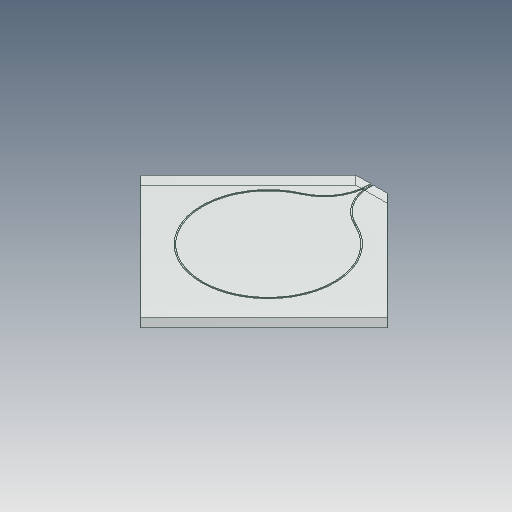
# Autodesk Inventor part: Scintillator Tile
Saved by Autodesk Inventor 2020 (Build 240168000, 168)
## iProperties
Created: 2015-08-14
Part Number: Scintillator Tile
Material: ABS Plastic
Document SubType Name: Modeling
Designer: Cosmic
Density: 1.06 g/cm^3
Appearance: Clear
Author: Cosmic
Autodesk Inventor part; units mm, degrees
note: some values were not read from the file. Chosen so that the rebuilt part matches the saved one: sketch regions of "Extrusion13". Left out: dimensions or parameters whose unit could not be read.
ref_plane "YZ Plane" through (0, 0, 0) normal (1, 0, 0) x (0, 1, 0)
ref_plane "XZ Plane" through (0, 0, 0) normal (0, 1, 0) x (-1, 0, 0)
ref_plane "XY Plane" through (0, 0, 0) normal (0, 0, 1) x (1, 0, 0)
sketch "Sketch11" plane through (0, 0, 0) normal (0, 0, 1) x (1, 0, 0)
  line L0 (0, -141.4214) -> (141.4214, 0)
  line L1 (141.4214, 0) -> (0, 141.4214)
  line L2 (0, 141.4214) -> (-141.4214, 0)
  line L3 (-141.4214, 0) -> (0, -141.4214)
  line L4 (0, -141.4214) -> (0, 141.4214) construction
  line L5 (141.4214, 0) -> (-141.4214, 0) construction
  line L6 (0, -141.4214) -> (200, -141.4214) construction
  point P0 (0, 0)
  dimension "d80" = 200
  dimension "d81" = 45
  dimension "d82" = 200
  constraints: 14 end point, 2 midpoint, 2 parallel, 1 equal length, 1 horizontal, 1 perpendicular
  measures "d80" distance of L0.start L0.end
  measures "d81" angle of L6 L0
  measures "d82" distance of L1.end L0.end
extrude "Extrusion12" add sketch "Sketch11" along normal blind 10
chamfer "Chamfer1" distance 25.4 angle 45 1 edges at (0, 141.4214, 5)
sketch "Sketch13" plane through (0, 0, 10) normal (0, 0, 1) x (1, 0, 0)
  line L0 (72.5, 123.4608) -> (-72.5, 123.4608)
  arc A0 (-30.4632, 73.5832) -> (30.4632, 73.5832) centre (0, 5.0485) ccw
  arc A1 (-30.9912, 74.7711) -> (-38.9161, 70.678) centre (0, 5.0485) ccw
  arc A2 (-30.9912, 74.7711) -> (-1.3, 120.4608) centre (-51.3, 120.4608) ccw
  arc A3 (30.9912, 74.7711) -> (80.4111, 79.8094) centre (51.3, 120.4608) ccw
  arc A4 (-38.9161, 70.678) -> (-30.4632, 73.5832) centre (-51.3, 120.4608) ccw
  arc A5 (22.6429, 77.9114) -> (30.4632, 73.5832) centre (51.3, 120.4608) ccw
  line L1 (-51.3, 120.4608) -> (51.3, 120.4608)
  arc A6 (-80.4111, 79.8094) -> (-30.9912, 74.7711) centre (-51.3, 120.4608) ccw
  arc A7 (-80.3294, 78.1644) -> (-38.9161, 70.678) centre (-51.3, 120.4608) ccw
  arc A8 (-1.3, 120.4608) -> (-80.4111, 79.8094) centre (-51.3, 120.4608) ccw
  arc A9 (-30.4632, 73.5832) -> (-22.6429, 77.9114) centre (-51.3, 120.4608) ccw
  arc A10 (30.4632, 73.5832) -> (-30.4632, 73.5832) centre (0, 5.0485) ccw
  arc A11 (-22.6429, 77.9114) -> (-30.9912, 74.7711) centre (0, 5.0485) ccw
  arc A12 (-38.9161, 70.678) -> (38.9161, 70.678) centre (0, 5.0485) ccw
  arc A13 (22.6429, 77.9114) -> (-22.6429, 77.9114) centre (0, 5.0485) ccw
  arc A14 (30.9912, 74.7711) -> (22.6429, 77.9114) centre (0, 5.0485) ccw
  arc A15 (0, 120.4608) -> (22.6429, 77.9114) centre (51.3, 120.4608) ccw
  arc A16 (1.3, 120.4608) -> (30.9912, 74.7711) centre (51.3, 120.4608) ccw
  arc A17 (0, 120.4608) -> (-80.3294, 78.1644) centre (-51.3, 120.4608) ccw
  arc A18 (-22.6429, 77.9114) -> (0, 120.4608) centre (-51.3, 120.4608) ccw
  arc A19 (30.4632, 73.5832) -> (38.9161, 70.678) centre (51.3, 120.4608) ccw
  arc A20 (38.9161, 70.678) -> (30.9912, 74.7711) centre (0, 5.0485) ccw
  arc A21 (38.9161, 70.678) -> (102.4649, 116.7406) centre (51.3, 120.4608) ccw
  arc A22 (80.4111, 79.8094) -> (1.3, 120.4608) centre (51.3, 120.4608) ccw
  arc A23 (102.4649, 116.7406) -> (0, 120.4608) centre (51.3, 120.4608) ccw
  line L2 (-17.9605, 123.4608) -> (17.9605, 123.4608) projected
  line L3 (-17.9605, 123.4608) -> (-141.4214, 0) projected
  line L4 (-141.4214, 0) -> (0, -141.4214) projected
  line L5 (0, -141.4214) -> (141.4214, 0) projected
  line L6 (141.4214, 0) -> (17.9605, 123.4608) projected
  point P0 (0, 0)
  point P1 (0, 0)
  point P2 (0, 120.4608)
  dimension "d97" = 1.3
  dimension "d98" = 1.3
  dimension "d99" = 1.3
  dimension "d100" = 100
  dimension "d101" = 100
  dimension "d102" = 150
  dimension "d103" = 3
  dimension "d111" = 17.9605
  dimension "d112" = 35.921
  constraints: 49 point on circle, 24 centre point, 4 end point, 3 tangent, 2 point on line, 1 collinear, 1 horizontal, 1 midpoint
  measures "d97" radial gap between concentric circles of A4 A2
  measures "d98" radial gap between concentric circles of A3 A5
  measures "d99" radial gap between concentric circles of A0 A1
  measures "d100" diameter of A2
  measures "d101" diameter of A3
  measures "d102" diameter of A0
  measures "d103" distance between parallel lines of L0 L1
  measures "d111" horizontal distance of A18.end L2.start
  measures "d112" distance of L2.start L2.end
extrude "Extrusion13" cut sketch "Sketch13" against normal blind 1.15 contours A16 A14 A15 L1 | A18 A11 A2 L1 | A15 A13 A18 | A20 A19 A5 A14 | A9 A4 A1 A11 | A12 A4 A0 A19
sketch "Sketch14" plane through (0, 0, 8.85) normal (0, 0, 1) x (1, 0, 0)
  arc A0 (-22.6429, 77.9114) -> (0, 120.4608) centre (-51.3, 120.4608) ccw projected
  arc A1 (0, 120.4608) -> (22.6429, 77.9114) centre (51.3, 120.4608) ccw projected
  arc A2 (22.6429, 77.9114) -> (-22.6429, 77.9114) centre (0, 5.0485) ccw projected
  point P0 (0, 0)
extrude "Extrusion14" add sketch "Sketch14" along normal up to surface (1.15 mm away)
sketch "Sketch15" plane through (-17.9605, 123.4608, 10) normal (0, 1, 0) x (1, 0, 0)
  line L0 (19.2605, 0) -> (19.2605, 1.15) projected
  line L1 (16.6605, 0) -> (16.6605, 1.15) projected
  line L2 (16.6605, 1.15) -> (17.9605, 1.15) projected
  line L3 (17.9605, 1.15) -> (19.2605, 1.15) projected
  line L4 (19.2605, 1.15) -> (48.9517, 1.15) projected
  line L5 (19.2605, 1.15) -> (16.6605, 1.15)
  line L6 (16.6605, 1.15) -> (16.6605, 0)
  line L7 (16.6605, 0) -> (19.2605, 0)
  line L8 (19.2605, 0) -> (19.2605, 1.15)
  point P0 (17.9605, 10)
  constraints: 8 end point, 2 parallel, 1 horizontal, 1 perpendicular
extrude "Extrusion15" cut sketch "Sketch15" against normal blind 9
fillet "Fillet2" radius 0.65 8 edges at (9.3748, 93.216, 8.85) (-4.4597, -71.121, 8.85) (-9.3748, 93.216, 8.85) (-1.3, 121.9608, 8.85) (1.3, 121.9608, 8.85) (0, -69.9515, 8.85) (-9.9961, 90.0358, 8.85) (9.9961, 90.0358, 8.85)
equation "\"d80\" = ScintillatorWidth"
equation "\"d82\" = ScintillatorHeight"
equation "\"d83\" = ScintillatorThickness"
equation "\"d85\" = cornerChamfer"
equation "\"d111\" = 0.5 * d112"
equation "\"d117\" = 3 * ScintillatorEdgeClearence"
equation "\"d119\" = OpticalFiberClearence + 0.5 * OpticalFiberDiameter"
equation "\"d5\" = OpticalFiberDiameter + 2 * OpticalFiberClearence"
equation "\"d21\" = d5"
equation "\"d22\" = d5"
equation "\"OpticalFiberDiameter\" = 1"
equation "\"ScintillatorThickness\" = 10"
equation "\"OpticalFiberClearence\" = 0.15"
equation "\"ScintillatorEdgeClearence\" = 3"
equation "\"ScintillatorWidth\" = 200"
equation "\"ScintillatorHeight\" = 200"
equation "\"LoopLargeTrackRatio\" = 1.5"
equation "\"cornerChamfer\" = 25.4"
equation "\"d106\" = 3"
equation "\"d107\" = 1"
equation "\"d108\" = 1.1"
equation "\"d109\" = 145"
equation "\"d110\" = 0.15"
equation "\"FiberEdgeOffsett\" = 5"
equation "\"FiberSensorClerence\" = 0.5"
equation "\"mountingSpacing\" = 18"
equation "\"silveringThickness\" = 0.2"
body "Solid1"
body "Solid2"
